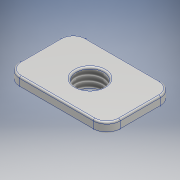
# Autodesk Inventor part: Noix M5
Saved by Autodesk Inventor 2017 (Build 210142000, 142)
## iProperties
Company: FABLAB Frenchmakers
Part Number: Noix M5
Material: Aluminium
Document SubType Name: Modeling
Designer: FABLAB Frenchmakers
Density: 2.7 g/cm^3
Appearance: Aluminium - Plat(2)
Mass: 0.614976 g
Surface Area: 3.88567 cm^2
Volume: 0.227769 cm^3
Stock Number: 1420-01-13
Project: 1420 Vauban 3D XL
Autodesk Inventor part; units mm, degrees
ref_plane "YZ Plane" through (0, 0, 0) normal (1, 0, 0) x (0, 1, 0)
ref_plane "XZ Plane" through (0, 0, 0) normal (0, 1, 0) x (-1, 0, 0)
ref_plane "XY Plane" through (0, 0, 0) normal (0, 0, 1) x (1, 0, 0)
sketch "Esquisse1" plane through (0, 0, 0) normal (0, 0, 1) x (1, 0, 0)
  line L0 (-7.5, -5) -> (7.5, -5)
  line L1 (7.5, -5) -> (7.5, 5)
  line L2 (7.5, 5) -> (-7.5, 5)
  line L3 (-7.5, 5) -> (-7.5, -5)
  line L4 (-7.5, -5) -> (7.5, 5) construction
  line L5 (7.5, -5) -> (-7.5, 5) construction
  point P0 (0, 0)
  dimension "d0" = 15
  dimension "d1" = 10
  constraints: 12 end point, 2 midpoint, 2 parallel, 1 horizontal, 1 perpendicular
  measures "d0" distance of L2.end L1.end
  measures "d1" distance of L1.end L0.end
extrude "Extrusion1" add sketch "Esquisse1" along normal blind 1.5
fillet "Congé1" radius 2 4 edges at (7.5, 5, 0.75) (-7.5, 5, 0.75) (7.5, -5, 0.75) (-7.5, -5, 0.75)
sketch "Esquisse2" plane through (0, 0, 0) normal (0, 0, 1) x (1, 0, 0)
  circle A0 centre (0, 0) radius 3.25
  dimension "d5" = 6.5
  constraints: 1 centre point, 1 coincident
  measures "d5" diameter of A0
extrude "Extrusion2" add sketch "Esquisse2" against normal blind 1.5
sketch "Esquisse3" plane through (0, 0, -1.5) normal (0, 0, -1) x (-1, 0, 0)
  point P0 (0, 0)
  point P1 (0, 0)
  constraints: 1 coincident
hole "Perçage1" at (0, 0, -1.5) direction (0, 0, 1) diameter 4.134 depth 14.2 tip angle 118 thread size "M5x0.8" class "6H" standard "ISO Metric profile"
fillet "Congé2" radius 0.25 20 edges at (6.9142, 4.4142, 0) (0, 5, 0) (-6.9142, 4.4142, 0) (-7.5, 0, 0) (-6.9142, -4.4142, 0) (0, -5, 0) (6.9142, -4.4142, 0) (7.5, 0, 0) (6.9142, 4.4142, 1.5) (0, 5, 1.5) (-6.9142, 4.4142, 1.5) (-7.5, 0, 1.5) (-6.9142, -4.4142, 1.5) (0, -5, 1.5) (6.9142, -4.4142, 1.5) (7.5, 0, 1.5) (-3.25, 0, 0) (-3.25, 0, -1.5) (0, -2.067, 1.5) (0, -2.067, -1.5)
